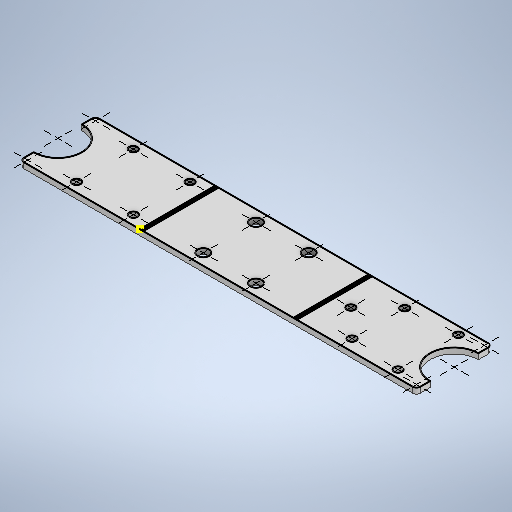
# Autodesk Inventor part: CAM_axis_2_bottom_frame
Saved by Autodesk Inventor 2025.2 (Build 292293000, 293)
## iProperties
Created: 2025-08-09
Part Number: CAM_axis_2_bottom_frame
Material: Generic
Document SubType Name: Modeling
Designer: User
Density: 1 g/cm^3
Appearance: Default
Author: User
Autodesk Inventor part; units mm, degrees
ref_plane "YZ Plane" through (0, 0, 0) normal (1, 0, 0) x (0, 1, 0)
ref_plane "XZ Plane" through (0, 0, 0) normal (0, 1, 0) x (-1, 0, 0)
ref_plane "XY Plane" through (0, 0, 0) normal (0, 0, 1) x (1, 0, 0)
sketch "Sketch1" plane through (0, 0, 0) normal (0, 1, 0) x (-1, 0, 0)
  line L0 (-41.2289, 0) -> (-41.2289, -20)
  line L1 (-0.4496, -20) -> (-0.4496, 0)
  circle A0 centre (4.19, -2.475) radius 1.05
  circle A1 centre (4.19, -17.525) radius 1.05
  circle A2 centre (19.29, -17.525) radius 1.05
  circle A3 centre (19.29, -2.475) radius 1.05
  circle A4 centre (-53.3486, -17) radius 1.05
  circle A5 centre (-46.0486, -10) radius 1.05
  circle A6 centre (-53.3486, -3) radius 1.05
  circle A7 centre (-66.5686, -2) radius 1.05
  circle A8 centre (-66.5686, -18) radius 1.05
  circle A9 centre (-27.8393, -17) radius 1.5
  circle A10 centre (-13.8393, -3) radius 1.5
  circle A11 centre (-27.8393, -3) radius 1.5
  circle A12 centre (-13.8393, -17) radius 1.5
  arc A13 (30.79, -20) -> (31.79, -19) centre (30.79, -19) ccw
  line L2 (31.79, -19) -> (31.79, -16.4)
  arc A14 (31.79, -1) -> (30.79, 0) centre (30.79, -1) ccw
  line L3 (31.79, -3.6) -> (31.79, -1)
  arc A15 (-72.4686, 0) -> (-73.4686, -1) centre (-72.4686, -1) ccw
  arc A16 (-73.4686, -19) -> (-72.4686, -20) centre (-72.4686, -19) ccw
  line L4 (-73.4686, -1) -> (-73.4686, -3.6)
  line L5 (-73.4686, -16.4) -> (-73.4686, -19)
  arc A17 (31.79, -3.6) -> (31.79, -16.4) centre (31.79, -10) ccw
  arc A18 (-73.4686, -16.4) -> (-73.4686, -3.6) centre (-73.4686, -10) ccw
  line L6 (30.79, -20) -> (-72.4686, -20)
  line L7 (-72.4686, 0) -> (30.79, 0)
  line L8 (-41.6786, -20) -> (-41.6786, 0)
  line L9 (-40.7793, 0) -> (-40.7793, -20)
  line L10 (-0.8993, -20) -> (-0.8993, 0)
  line L11 (0, 0) -> (0, -20)
  constraints: 24 end point, 19 centre point, 15 equal radius, 12 point on circle, 12 point on line, 12 tangent, 10 vertical, 7 parallel, 2 horizontal, 2 perpendicular, 63 other
extrude "Extrusion1" add sketch "Sketch1" against normal blind 1.5
body "Solid1"
